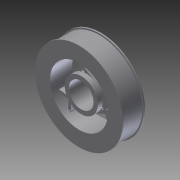
# Autodesk Inventor part: new weel hub
Saved by Autodesk Inventor 2012 (Build 160160000, 160)
## iProperties
Created: 2012-08-10
Part Number: new weel hub
Material: Default
Document SubType Name: Modeling
Designer: Bryce
Density: 1 g/cm^3
Author: Bryce
Autodesk Inventor part; units mm, degrees
ref_plane "YZ Plane" through (0, 0, 0) normal (1, 0, 0) x (0, 1, 0)
ref_plane "XZ Plane" through (0, 0, 0) normal (0, 1, 0) x (-1, 0, 0)
ref_plane "XY Plane" through (0, 0, 0) normal (0, 0, 1) x (1, 0, 0)
sketch "Sketch1" plane through (0, 0, 0) normal (0, 0, 1) x (1, 0, 0)
  circle A0 centre (0, 0) radius 50.8
  circle A1 centre (0, 0) radius 19.05
  circle A2 centre (0, 0) radius 49.2125
  circle A3 centre (0, 0) radius 33.3375
  line L0 (19.05, 0) -> (22.61, -8.1654) construction
  circle A4 centre (0, 0) radius 14.2875
  line L1 (0, 0) -> (14.6542, -12.172) construction
  line L2 (0, 0) -> (19.05, 0) construction
  line L3 (14.6542, -12.172) -> (22.61, -8.1654) construction
  line L4 (22.61, -8.1654) -> (33.2177, -2.8233) construction
  line L5 (22.61, -8.1654) -> (27.3567, -19.0526) construction
  line L6 (-9.525, 16.4978) -> (-4.2335, 23.6635) construction
  line L7 (0, 0) -> (3.2142, 18.7769) construction
  line L8 (0, 0) -> (-9.525, 16.4978) construction
  line L9 (3.2142, 18.7769) -> (-4.2335, 23.6635) construction
  line L10 (-4.2335, 23.6635) -> (-14.1638, 30.1791) construction
  line L11 (-4.2335, 23.6635) -> (2.8217, 33.2179) construction
  line L12 (-9.525, -16.4978) -> (-18.3764, -15.4981) construction
  line L13 (0, 0) -> (-17.8683, -6.6049) construction
  line L14 (0, 0) -> (-9.525, -16.4978) construction
  line L15 (-17.8683, -6.6049) -> (-18.3764, -15.4981) construction
  line L16 (-18.3764, -15.4981) -> (-19.0539, -27.3557) construction
  line L17 (-18.3764, -15.4981) -> (-30.1784, -14.1652) construction
  line L18 (17.4625, 7.6134) -> (28.3964, -17.4652)
  line L19 (18.7605, -3.3083) -> (26.2679, -20.5277)
  line L20 (8.5684, -17.0142) -> (33.0033, -4.7088)
  line L21 (16.5453, -9.4421) -> (33.3227, -0.993)
  line L22 (-17.5213, -28.3618) -> (-16.4498, -9.6076)
  line L23 (-20.5795, -26.2273) -> (-19.019, 1.0866)
  line L24 (-29.3235, -15.8594) -> (-2.1379, -18.9297)
  line L25 (-30.9114, -12.4849) -> (-12.2453, -14.593)
  line L26 (4.6435, 33.0125) -> (-6.5152, 17.9012)
  line L27 (0.9271, 33.3246) -> (-15.3246, 11.3163)
  line L28 (-12.4237, 30.9361) -> (10.4505, 15.9276)
  line L29 (-15.8014, 29.3548) -> (-0.0955, 19.0498)
  point P0 (-17.7936, -6.8036)
  dimension "d1" = 38.1
  dimension "d3" = 66.675
  dimension "d0" = 101.6
  dimension "d2" = 98.425
  dimension "d71" = 28.575
  dimension "d81" = 8.9077
  dimension "d82" = 11.877
  dimension "d83" = 8.9077
  dimension "d84" = 11.877
  dimension "d87" = 360
  dimension "d91" = 1.5875
  dimension "d92" = 1.5875
  dimension "d96" = 1.5875
  dimension "d97" = 1.5875
  dimension "d99" = 1.5875
  dimension "d100" = 1.5875
  dimension "d101" = 1.5875
  dimension "d103" = 1.5875
  constraints: 60 end point, 12 parallel, 6 coincident, 3 centre point, 2 collinear, 1 horizontal, 1 horizontal alignment, 76 other
  measures "d0" diameter of A0
  measures "d2" diameter of A2
  measures "d71" diameter of A4
  measures "d81" distance of L1.end L0.end
  measures "d82" distance of L0.end L4.end
  measures "d83" distance of L0.start L0.end
  measures "d84" distance of L0.end L5.end
  measures "d91" distance between parallel lines of L3 L21
  measures "d92" distance between parallel lines of L3 L20
  measures "d96" distance between parallel lines of L0 L19
  measures "d97" distance between parallel lines of L18 L0
  measures "d99" distance between parallel lines of L16 L22
  measures "d100" distance between parallel lines of L17 L25
  measures "d101" distance between parallel lines of L6 L26
  measures "d103" distance between parallel lines of L10 L29
extrude "Extrusion1" add sketch "Sketch1" along normal mid plane 20.32 contours A1
extrude "Extrusion2" add sketch "Sketch1" along normal mid plane 25.4 contours A2
extrude "Extrusion3" add sketch "Sketch1" along normal mid plane 25.4 contours A0
extrude "Extrusion4" cut sketch "Sketch1" along normal mid plane 22.225 contours A0
extrude "Extrusion6" add sketch "Sketch1" along normal mid plane 9.525 contours A1 L18 L21 L19 | A1 L29 L26 L28 | L21 A3 L20 L18 | L18 L20 L19 L21 | L21 L19 L20 A1 | L28 L27 A3 L26 | L26 L29 L27 L28 | L18 A3 L19 L20 | A1 L27 L29 L26 | L27 L29 A3 L28 | L24 L22 L25 A1 | L24 L23 L25 L22 | L22 A3 L23 L24 | A1 L22 L25 L23 | L24 A3 L25 L23
fillet "Fillet3" radius 0.7937 30 edges at (33.0033, -4.7088, 0) (28.3964, -17.4652, 0) (24.6654, -8.9077, 0) (33.3227, -0.993, 0) (26.2679, -20.5277, 0) (16.5453, -9.4421, 0) (21.8254, -10.338, 0) (23.3946, -5.9928, 0) (20.5545, -7.4231, 0) (18.7605, -3.3083, 0) (-12.2453, -14.593, 0) (-16.4498, -9.6076, 0) (-16.7059, -14.0892, 0) (-17.5213, -28.3618, 0) (-20.5795, -26.2273, 0) (-20.047, -16.907, 0) (-29.3235, -15.8594, 0) (-30.9114, -12.4849, 0) (-6.5152, 17.9012, 0) (-0.0955, 19.0498, 0) (-3.8487, 21.5123, 0) (-16.8872, -17.2639, 0) (-19.8657, -13.7323, 0) (-6.5074, 23.2567, 0) (-4.6184, 25.8148, 0) (-1.9597, 24.0703, 0) (-12.4237, 30.9361, 0) (0.9271, 33.3246, 0) (4.6435, 33.0125, 0) (-15.8014, 29.3548, 0)
body "Solid1"
